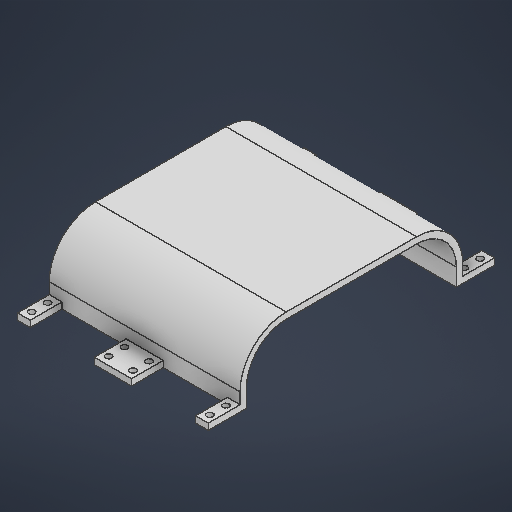
# Autodesk Inventor part: back
Saved by Autodesk Inventor 2026.1 (Build 301233000, 233)
## iProperties
Created: 2025-11-04
Part Number: back
Material: Generic
Document SubType Name: Modeling
Designer: emanuel
Density: 1 g/cm^3
Appearance: Default
Author: emanuel
Autodesk Inventor part; units mm, degrees
ref_plane "YZ Plane" through (0, 0, 0) normal (1, 0, 0) x (0, 1, 0)
ref_plane "XZ Plane" through (0, 0, 0) normal (0, 1, 0) x (-1, 0, 0)
ref_plane "XY Plane" through (0, 0, 0) normal (0, 0, 1) x (1, 0, 0)
sketch "Sketch1" plane through (0, 0, 0) normal (1, 0, 0) x (0, 1, 0)
  line L0 (0, 0) -> (40, 0)
  line L1 (40, 0) -> (40, -180)
  line L2 (40, -180) -> (0, -180)
  line L3 (0, -180) -> (0, 0)
  line L4 (0, 0) -> (4, 0)
  line L5 (4, 0) -> (4, -20)
  line L6 (4, -20) -> (0, -20)
  line L7 (0, -20) -> (0, 0)
  line L8 (0, -180) -> (4, -180)
  line L9 (4, -180) -> (4, -160)
  line L10 (4, -160) -> (0, -160)
  line L11 (0, -160) -> (0, -180)
  line L12 (4, -20) -> (4, -56)
  line L13 (4, -160) -> (4, -124)
  line L14 (4, -56) -> (40, -56)
  line L15 (4, -124) -> (40, -124)
  line L16 (40, -124) -> (4, -160)
  line L17 (4, -20) -> (40, -56)
  line L18 (40, -56) -> (36, -56)
  line L19 (36, -56) -> (36, -124)
  line L20 (36, -124) -> (40, -124)
  line L21 (40, -124) -> (40, -56)
  line L22 (4, -20) -> (1.1716, -22.8284)
  line L23 (1.1716, -22.8284) -> (36, -57.6569)
  line L24 (1.1716, -22.8284) -> (0, -21.6569)
  line L25 (4, -160) -> (1.1716, -157.1716)
  line L26 (1.1716, -157.1716) -> (36, -122.3431)
  line L27 (1.1716, -157.1716) -> (-0.2426, -158.5858)
  line L28 (0, -20) -> (40, -20)
  line L29 (40, -20) -> (40, -24)
  line L30 (40, -24) -> (0, -24)
  line L31 (0, -24) -> (0, -20)
  line L32 (40, -20) -> (36, -20)
  line L33 (36, -20) -> (36, -56)
  line L34 (36, -56) -> (40, -56)
  line L35 (40, -56) -> (40, -20)
  line L36 (0, -160) -> (40, -160)
  line L37 (40, -160) -> (40, -156)
  line L38 (40, -156) -> (0, -156)
  line L39 (0, -156) -> (0, -160)
  line L40 (40, -160) -> (36, -160)
  line L41 (36, -160) -> (36, -124)
  line L42 (36, -124) -> (40, -124)
  line L43 (40, -124) -> (40, -160)
  point P0 (0, -158.3431)
  point P1 (36, -156)
  point P2 (36, -24)
  dimension "d0" = 40
  dimension "d1" = 180
  dimension "d2" = 4
  dimension "d3" = 20
  dimension "d4" = 4
  dimension "d5" = 20
  dimension "d6" = 36
  dimension "d7" = 36
  dimension "d8" = 4
  dimension "d9" = 4
  dimension "d10" = 4
  dimension "d67" = 40
  dimension "d68" = 4
  dimension "d69" = 40
  dimension "d70" = 4
  constraints: 88 end point, 17 parallel, 12 perpendicular, 8 horizontal, 6 point on line, 2 vertical
  measures "d0" distance of L1.end L2.end
  measures "d1" distance of L0.end L1.end
  measures "d2" distance of L5.end L6.end
  measures "d3" distance of L4.end L5.end
  measures "d4" distance of L10.end L9.end
  measures "d5" distance of L9.end L8.end
  measures "d6" distance of L5.end L12.end
  measures "d7" distance of L9.end L13.end
  measures "d8" distance of L20.end L19.end
  measures "d9" distance of L5.end L22.end
  measures "d10" distance of L9.end L25.end
  measures "d67" distance of L29.end L30.end
  measures "d68" distance of L28.end L29.end
  measures "d69" distance of L38.end L37.end
  measures "d70" distance of L37.end L36.end
extrude "Extrusion1" add sketch "Sketch1" along normal blind 120 contours L0 L5 L6 L3 | L6 L22 L24 L3 | L17 L30 L12 | L28 L33 L30 L17 | L12 L30 L23 L22 | L24 L23 L30 L3 | L1 L30 L33 L28 | L1 L17 L33 L30 | L17 L14 L33 | L38 L26 L27 L3 | L1 L15 L19 L14 | L27 L25 L10 L3 | L38 L13 L25 L26 | L16 L41 L15 | L1 L38 L41 L16 | L10 L9 L2 L3 | L38 L16 L13 | L1 L36 L41 L38 | L16 L38 L41 L36
sketch "Sketch2" plane through (0, 4, 0) normal (0, 1, 0) x (1, 0, 0)
  line L0 (0, 0) -> (120, 0) projected
  line L1 (0, 0) -> (4, 0)
  line L2 (4, 0) -> (4, 5)
  line L3 (4, 5) -> (0, 5)
  line L4 (0, 5) -> (0, 0)
  line L5 (4, 5) -> (4, 15)
  circle A0 centre (4, 15) radius 2
  circle A1 centre (4, 5) radius 2
  line L6 (120, 0) -> (116, 0)
  line L7 (116, 0) -> (116, 5)
  line L8 (116, 5) -> (120, 5)
  line L9 (120, 5) -> (120, 0)
  line L10 (116, 5) -> (116, 15)
  circle A2 centre (116, 15) radius 2
  circle A3 centre (116, 5) radius 2
  line L11 (0, 20) -> (120, 20) projected
  line L12 (120, 0) -> (112, 0)
  line L13 (112, 0) -> (112, 20)
  line L14 (112, 20) -> (120, 20)
  line L15 (120, 20) -> (120, 0)
  line L16 (0, 0) -> (8, 0)
  line L17 (8, 0) -> (8, 20)
  line L18 (8, 20) -> (0, 20)
  line L19 (0, 20) -> (0, 0)
  line L20 (112, 20) -> (71.7, 20)
  line L21 (71.7, 20) -> (71.7, 0)
  line L22 (71.7, 0) -> (112, 0)
  line L23 (112, 0) -> (112, 20)
  line L24 (8, 20) -> (48.3, 20)
  line L25 (48.3, 20) -> (48.3, 0)
  line L26 (48.3, 0) -> (8, 0)
  line L27 (8, 0) -> (8, 20)
  line L28 (48.3, 0) -> (52.3, 0)
  line L29 (52.3, 0) -> (52.3, 5)
  line L30 (52.3, 5) -> (48.3, 5)
  line L31 (48.3, 5) -> (48.3, 0)
  line L32 (52.3, 5) -> (52.3, 15)
  circle A4 centre (52.3, 15) radius 2
  circle A5 centre (52.3, 5) radius 2
  line L33 (48.3, 20) -> (48.3, 0)
  line L34 (71.7, 0) -> (67.7, 0)
  line L35 (67.7, 0) -> (67.7, 5)
  line L36 (67.7, 5) -> (71.7, 5)
  line L37 (71.7, 5) -> (71.7, 0)
  line L38 (67.7, 5) -> (67.7, 15)
  circle A6 centre (67.7, 15) radius 2
  circle A7 centre (67.7, 5) radius 2
  line L39 (71.7, 20) -> (71.7, 0)
  line L40 (0, 20) -> (120, 20)
  line L41 (120, 20) -> (120, 0)
  line L42 (120, 0) -> (0, 0)
  line L43 (0, 0) -> (0, 20)
  line L44 (0, 180) -> (0, 160) projected
  line L45 (0, 180) -> (-1.8149, 180)
  line L46 (0, 160) -> (4, 160)
  line L47 (4, 160) -> (4, 165)
  line L48 (4, 165) -> (0, 165)
  line L49 (0, 165) -> (0, 160)
  line L50 (4, 165) -> (4, 175)
  circle A8 centre (4, 175) radius 2
  circle A9 centre (4, 165) radius 2
  line L51 (120, 160) -> (116, 160)
  line L52 (116, 160) -> (116, 165)
  line L53 (116, 165) -> (120, 165)
  line L54 (120, 165) -> (120, 160)
  line L55 (116, 165) -> (116, 175)
  circle A10 centre (116, 175) radius 2
  circle A11 centre (116, 165) radius 2
  line L56 (120, 160) -> (112, 160)
  line L57 (112, 160) -> (112, 180)
  line L58 (112, 180) -> (120, 180)
  line L59 (120, 180) -> (120, 160)
  line L60 (0, 160) -> (8, 160)
  line L61 (8, 160) -> (8, 180)
  line L62 (8, 180) -> (0, 180)
  line L63 (0, 180) -> (0, 160)
  line L64 (112, 180) -> (71.7, 180)
  line L65 (71.7, 180) -> (71.7, 160)
  line L66 (71.7, 160) -> (112, 160)
  line L67 (112, 160) -> (112, 180)
  line L68 (8, 180) -> (48.3, 180)
  line L69 (48.3, 180) -> (48.3, 160)
  line L70 (48.3, 160) -> (8, 160)
  line L71 (8, 160) -> (8, 180)
  line L72 (52.3, 165) -> (52.3, 175)
  circle A12 centre (52.3, 165) radius 2
  circle A13 centre (52.3, 175) radius 2
  line L73 (48.3, 180) -> (48.3, 160)
  line L74 (52.3, 165) -> (48.3, 165)
  line L75 (48.3, 160) -> (52.3, 160)
  line L76 (48.3, 165) -> (48.3, 160)
  line L77 (52.3, 160) -> (52.3, 165)
  line L78 (67.7, 160) -> (67.7, 165)
  line L79 (67.7, 165) -> (67.7, 175)
  circle A14 centre (67.7, 165) radius 2
  circle A15 centre (67.7, 175) radius 2
  line L80 (71.7, 160) -> (67.7, 160)
  line L81 (71.7, 165) -> (71.7, 160)
  line L82 (67.7, 165) -> (71.7, 165)
  line L83 (71.7, 180) -> (71.7, 160)
  line L84 (0, 180) -> (120, 180)
  line L85 (120, 180) -> (120, 160)
  line L86 (120, 160) -> (0, 160)
  line L87 (0, 160) -> (0, 180)
  dimension "d13" = 4
  dimension "d14" = 5
  dimension "d15" = 10
  dimension "d16" = 4
  dimension "d17" = 4
  dimension "d18" = 4
  dimension "d19" = 5
  dimension "d20" = 10
  dimension "d21" = 4
  dimension "d22" = 4
  dimension "d23" = 8
  dimension "d24" = 8
  dimension "d25" = 40.3
  dimension "d26" = 40.3
  dimension "d27" = 4
  dimension "d28" = 5
  dimension "d29" = 10
  dimension "d30" = 4
  dimension "d31" = 4
  dimension "d32" = 4
  dimension "d33" = 5
  dimension "d34" = 10
  dimension "d35" = 4
  dimension "d36" = 4
  dimension "d37" = 4
  dimension "d38" = 5
  dimension "d39" = 10
  dimension "d40" = 4
  dimension "d41" = 4
  dimension "d42" = 4
  dimension "d43" = 5
  dimension "d44" = 10
  dimension "d45" = 4
  dimension "d46" = 4
  dimension "d47" = 8
  dimension "d48" = 8
  dimension "d49" = 40.3
  dimension "d50" = 40.3
  dimension "d51" = 4
  dimension "d52" = 5
  dimension "d53" = 10
  dimension "d54" = 4
  dimension "d55" = 4
  dimension "d56" = 4
  dimension "d57" = 5
  dimension "d58" = 10
  dimension "d59" = 4
  dimension "d60" = 4
  constraints: 170 end point, 36 parallel, 19 horizontal, 18 perpendicular, 16 centre point, 16 coincident, 8 vertical, 4 point on line
  measures "d13" distance of L3.end L2.end
  measures "d14" distance of L2.end L1.end
  measures "d15" distance of L2.end L5.end
  measures "d16" diameter of A0
  measures "d17" diameter of A1
  measures "d18" distance of L7.end L8.end
  measures "d19" distance of L6.end L7.end
  measures "d20" distance of L7.end L10.end
  measures "d21" diameter of A2
  measures "d22" diameter of A3
  measures "d23" distance of L13.end L14.end
  measures "d24" distance of L18.end L17.end
  measures "d25" distance of L22.end L21.end
  measures "d26" distance of L25.end L26.end
  measures "d27" distance of L30.end L32.start
  measures "d28" distance of L32.start L28.end
  measures "d29" distance of L32.start L32.end
  measures "d30" diameter of A4
  measures "d31" diameter of A5
  measures "d32" distance of L35.end L37.start
  measures "d33" distance of L35.start L35.end
  measures "d34" distance of L35.end L38.end
  measures "d35" diameter of A6
  measures "d36" diameter of A7
  measures "d37" distance of L48.end L50.start
  measures "d38" distance of L50.start L47.start
  measures "d39" distance of L50.start L50.end
  measures "d40" diameter of A8
  measures "d41" diameter of A9
  measures "d42" distance of L52.end L53.end
  measures "d43" distance of L51.end L52.end
  measures "d44" distance of L52.end L55.end
  measures "d45" diameter of A10
  measures "d46" diameter of A11
  measures "d47" distance of L58.start L59.start
  measures "d48" distance of L62.end L61.end
  measures "d49" distance of L66.end L65.end
  measures "d50" distance of L70.start L71.start
  measures "d51" distance of L76.start L72.start
  measures "d52" distance of L72.start L77.start
  measures "d53" distance of L72.start L72.end
  measures "d54" diameter of A13
  measures "d55" diameter of A12
  measures "d56" distance of L78.end L82.end
  measures "d57" distance of L78.start L78.end
  measures "d58" distance of L78.end L79.end
  measures "d59" diameter of A15
  measures "d60" diameter of A14
extrude "Extrusion2" cut sketch "Sketch2" against normal blind 120 contours L17 L11 L25 L0 | A1 L3 L2 | L2 L5 A1 | A1 L5 L3 | A5 L30 L29 | L29 L32 A5 | A5 L32 L30 | L11 L13 L0 L21 | A7 L38 L35 | L35 L36 A7 | L38 A7 L36 | A3 L10 L7 | L7 L8 A3 | L8 L10 A3 | A0 | A2 | A4 | A6 | L68 L69 L70 L61 | A9 L50 L48 | L48 L47 A9 | L50 A9 L47 | L64 L57 L66 L65 | L74 L77 A12 | A12 L72 L74 | L77 L72 A12 | L82 L79 A14 | A14 L78 L82 | A14 L79 L78 | A11 L55 L52 | L52 L53 A11 | L53 L55 A11 | A8 | A10 | A13 | A15
fillet "Fillet1" radius 25 2 edges at (60, 36, -24) (60, 36, -156)
fillet "Fillet2" radius 29 2 edges at (60, 40, -20) (60, 40, -160)
body "Solid1"
